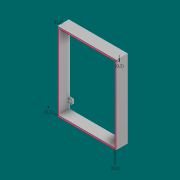
# Autodesk Inventor part: Struttura_intera
Saved by Autodesk Inventor 2020 (Build 240168000, 168)
## iProperties
Created: 2025-01-02
Part Number: Struttura_intera
Material: Plastica ABS
Document SubType Name: Modeling
Designer: Nicola Milia
Density: 1.06 g/cm^3
Appearance: Liscia - Bianco
Author: Nicola Milia
## iProperties of the stored document _Stampa 3D.ipt
Created: 2025-01-02
Part Number: _Stampa 3D
Material: Generico
Document SubType Name: Modeling
Designer: Nicola Milia
Density: 1 g/cm^3
Appearance: Default
Author: Nicola Milia
Autodesk Inventor part; units mm, degrees
ref_plane "YZ Plane" through (0, 0, 0) normal (1, 0, 0) x (0, 1, 0)
ref_plane "XZ Plane" through (0, 0, 0) normal (0, 1, 0) x (-1, 0, 0)
sketch "Schizzo1" plane through (0, 0, 0) normal (0, 0, 1) x (1, 0, 0)
  point P0 (0, 0)
sketch "Schizzo2" plane through (0, 0, 0) normal (0, 0, 1) x (1, 0, 0)
  line L0 (0, -121) -> (90, -121) projected
  line L1 (90, -121) -> (90, 0) projected
  line L2 (0, 0) -> (0, -121) projected
  line L3 (90, 0) -> (0, 0) projected
  circle A0 centre (86, -106) radius 2 projected
  circle A1 centre (4, -106) radius 2 projected
  circle A2 centre (4, -6) radius 2 projected
  circle A3 centre (86, -6) radius 2 projected
  line L4 (92, 2) -> (92, -123)
  line L5 (92, -123) -> (-2, -123)
  line L6 (-2, -123) -> (-2, 2)
  line L7 (-2, 2) -> (92, 2)
  dimension "d0" = 2
  constraints: 8 end point, 3 other
  measures "d0" distance between parallel lines of L1 L4
extrude "Estrusione1" add sketch "Schizzo2" along normal blind 18 contours L4 L5 L6 L7
ref_plane "Piano di lavoro1" through (45, -60.5, 1) normal (0, 0, 1) x (1, 0, 0)
sketch "Schizzo3" plane through (45, -60.5, 1) normal (0, 0, 1) x (1, 0, 0)
  circle A0 centre (41, -45.5) radius 2 projected
  circle A1 centre (-41, -45.5) radius 2 projected
  circle A2 centre (41, 54.5) radius 2 projected
  circle A3 centre (-41, 54.5) radius 2 projected
  line L0 (45, -60.5) -> (45, 60.5) projected
  line L1 (45, 60.5) -> (-45, 60.5) projected
  line L2 (-45, -60.5) -> (45, -60.5) projected
  line L3 (-45, 60.5) -> (-45, -60.5) projected
  line L4 (-45, -60.5) -> (-45, 60.5) projected
  line L5 (-39, -41.5) -> (-45, -41.5)
  line L6 (-45, -41.5) -> (-45, -49.5)
  line L7 (-45, -49.5) -> (-39, -49.5)
  line L8 (-37, -47.5) -> (-37, -43.5)
  arc A4 (-37, -43.5) -> (-39, -41.5) centre (-39, -43.5) ccw
  arc A5 (-39, -49.5) -> (-37, -47.5) centre (-39, -47.5) ccw
  line L9 (39, -41.5) -> (45, -41.5)
  line L10 (45, -41.5) -> (45, -49.5)
  line L11 (45, -49.5) -> (39, -49.5)
  line L12 (37, -47.5) -> (37, -43.5)
  arc A6 (37, -47.5) -> (39, -49.5) centre (39, -47.5) ccw
  arc A7 (39, -41.5) -> (37, -43.5) centre (39, -43.5) ccw
  line L13 (37, 60.5) -> (37, 52.5)
  line L14 (39, 50.5) -> (45, 50.5)
  line L15 (45, 50.5) -> (45, 60.5)
  arc A8 (37, 52.5) -> (39, 50.5) centre (39, 52.5) ccw
  line L16 (-45, 60.5) -> (-45, 50.5)
  line L17 (-45, 50.5) -> (-37, 50.5)
  line L18 (-37, 50.5) -> (-37, 60.5)
  point P0 (-45, -41.5)
  point P1 (-45, -49.5)
  point P2 (45, 50.5)
  constraints: 28 end point, 10 point on circle, 10 tangent, 6 parallel, 5 centre point, 4 perpendicular, 4 point on line, 2 equal radius
extrude "Estrusione2" add sketch "Schizzo3" along normal blind 2 contours L11 A6 L12 A7 L9 L0 | L3 L5 A4 L8 A5 L7 | L14 A8 L13 L1 L0 | L3 L1 L18 L17
fillet "Raccordo1" radius 2 1 edges at (8, -10, 2)
sketch "Schizzo4" plane through (0, 0, 0) normal (0, 0, -1) x (-1, 0, 0)
  line L0 (-90, 0) -> (-90, -121) projected
  line L1 (0, 0) -> (-90, 0) projected
  line L2 (0, -121) -> (0, 0) projected
  line L3 (-90, -121) -> (0, -121) projected
extrude "Estrusione3" cut sketch "Schizzo4" against normal blind 1.6
move faces "Sposta1" translate (0.4, 0, 0) faces at (90, -74.3333, 13)
move faces "Sposta2" translate (0, -0.25, 0) faces at (60.2667, -121, 6)
move faces "Sposta3" translate (0, 0.5, 0) faces at (57.4667, 0, 13)
move faces "Sposta4" translate (0.5, 0, 0) faces at (0, -74.25, 13)
move faces "Sposta5" translate (0, 0.25, 0) faces at (60.4333, -121.25, 6)
move faces "Sposta6" translate (-0.5, 0, 0) faces at (0.5, -74.1667, 13)
move faces "Sposta7" translate (0, -0.5, 0) faces at (57.4667, 0.5, 13)
move faces "Sposta8" translate (-0.4, 0, 0) faces at (90.4, -74.3333, 13) (-1.3333, -80.6667, 0)
sketch "Schizzo7" plane through (0, 0, 18) normal (0, 0, 1) x (1, 0, 0)
  line L0 (92, -123) -> (92, 2) projected
  line L1 (92, 2) -> (-2, 2) projected
  line L2 (-2, 2) -> (-2, -123) projected
  line L3 (-2, -123) -> (92, -123) projected
  line L4 (90, 0) -> (90, -121) projected
  line L5 (90, -121) -> (0, -121) projected
  line L6 (0, -121) -> (0, 0) projected
  line L7 (0, 0) -> (90, 0) projected
  dimension "d49" = 2
  dimension "d50" = 2
  dimension "d51" = 2
  dimension "d52" = 2
  measures "d49" horizontal distance of L0.end L4.start
  measures "d50" horizontal distance of L6.end L1.end
  measures "d51" horizontal distance of L0.start L4.end
  measures "d52" horizontal distance of L2.end L5.end
move faces "Sposta9" translate (0, 0, -0.4) faces at (91.3333, -80.6667, 0)
move faces "Sposta10" translate (0, 0, 0.6) faces at (0.6667, -106, 3) (4.0804, -1.3382, 3) (85.9196, -1.3382, 3) (89.3333, -106, 3)
sketch "Schizzo10" plane through (92, -123, -0.4) normal (0, 0, -1) x (-1, 0, 0)
  line L0 (0, 0) -> (0, 125) projected
  line L1 (94, 0) -> (0, 0) projected
  line L2 (94, 125) -> (94, 0) projected
  line L3 (0, 125) -> (94, 125) projected
  line L4 (2, 123) -> (2, 2) projected
  line L5 (92, 123) -> (2, 123) projected
  line L6 (92, 2) -> (92, 123) projected
  line L7 (2, 2) -> (92, 2) projected
  line L8 (92.5, 1.5) -> (92.5, 123.5)
  line L9 (92.5, 123.5) -> (1.5, 123.5)
  line L10 (1.5, 123.5) -> (1.5, 1.5)
  line L11 (1.5, 1.5) -> (92.5, 1.5)
  dimension "d61" = 0.5
  constraints: 8 end point, 3 other
  measures "d61" distance between parallel lines of L7 L11
extrude "Estrusione4" cut sketch "Schizzo10" against normal up to surface (2 mm away) contours L11 L10 L9 L8
